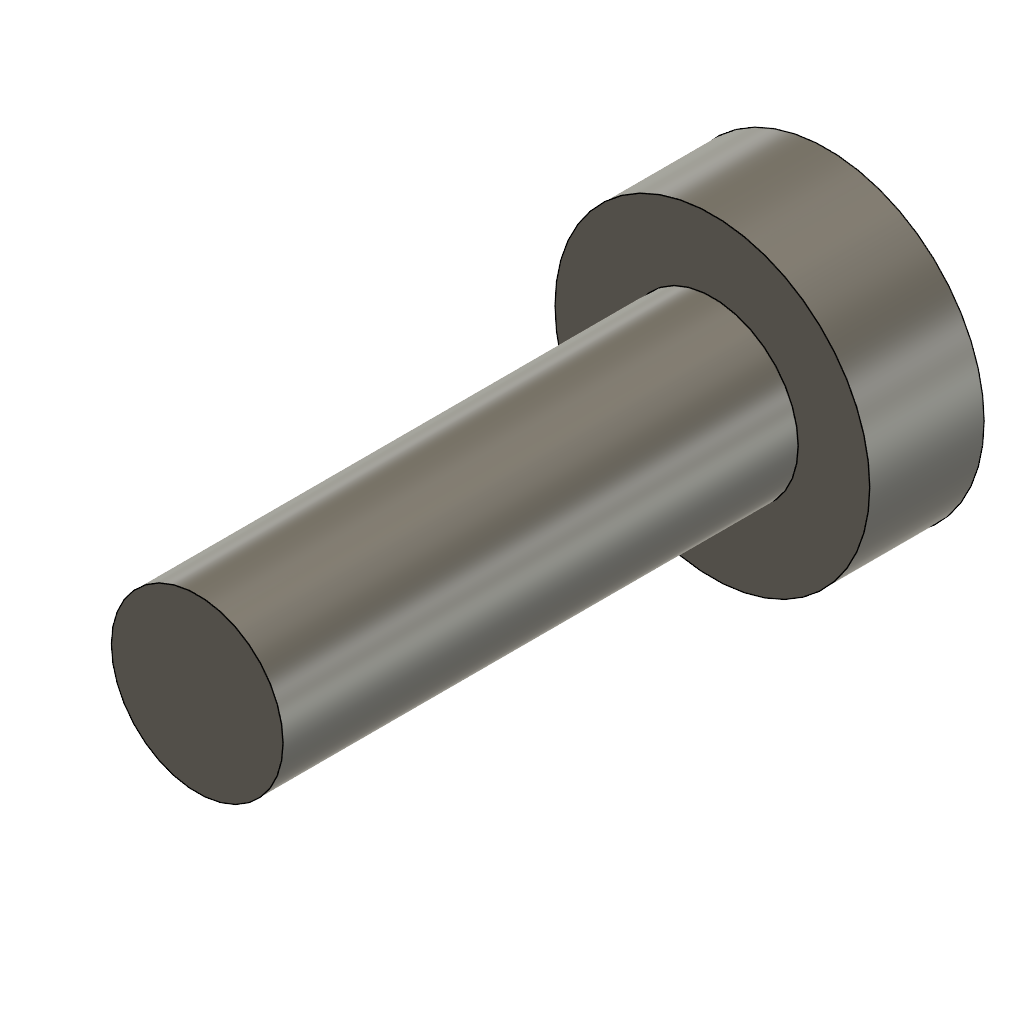
side_heat_rivet_print_2 (Autodesk Fusion 360 design; units mm, degrees)
part number: 2026-10-03-14-02-03-815
Autodesk Fusion 360 part; units mm, degrees
ref_plane "工作平面1" through (0, 0, 0) normal (0, 0, 1) x (1, 0, 0)
sketch "草图1" plane through (0, 0, 0) normal (0, 0, 1) x (1, 0, 0)
  circle A0 centre (0, 0) radius 2.75
extrude "Rivet flange 5.5 x 2 mm" add sketch "草图1" along normal blind 2
ref_plane "工作平面2" through (0, 0, 2) normal (0, 0, 1) x (1, 0, 0)
sketch "草图2" plane through (0, 0, 2) normal (0, 0, 1) x (1, 0, 0)
  circle A0 centre (0, 0) radius 1.5
extrude "3 mm rivet shank through ear and metal tab" add sketch "草图2" along normal blind 9
